Autodesk Inventor part; units mm, degrees
(part 2 of 2)
  spline S257 degree 2 poles (-118.3929, 389.4341) (-118.546, 389.3872) (-118.7461, 389.1921) (-118.7461, 389.0192) knots 0 0 0 1 2 2 2
  spline S258 degree 2 poles (-118.7461, 389.0192) (-118.7461, 388.8216) (-118.5238, 388.6215) (-118.3114, 388.6215) knots 0 0 0 1 2 2 2
  spline S259 degree 2 poles (-118.3114, 388.6215) (-118.1311, 388.6215) (-117.8347, 388.7771) (-117.7062, 388.8932) knots 0 0 0 1 2 2 2
  spline S260 degree 2 poles (-116.0884, 388.2856) (-116.402, 388.2856) (-116.7553, 388.6437) (-116.7553, 389.0315) knots 0 0 0 1 2 2 2
  line L211 (-116.7553, 389.0315) -> (-116.7553, 390.2986)
  line L212 (-116.7553, 390.2986) -> (-117.0146, 390.2986)
  line L213 (-117.0146, 390.2986) -> (-117.0146, 390.6173)
  line L214 (-117.0146, 390.6173) -> (-116.7553, 390.6173)
  line L215 (-116.7553, 390.6173) -> (-116.7553, 391.2743)
  line L216 (-116.7553, 391.2743) -> (-116.3699, 391.2743)
  line L217 (-116.3699, 391.2743) -> (-116.3699, 390.6173)
  line L218 (-116.3699, 390.6173) -> (-115.661, 390.6173)
  line L219 (-115.661, 390.6173) -> (-115.661, 390.2986)
  line L220 (-115.661, 390.2986) -> (-116.3699, 390.2986)
  line L221 (-116.3699, 390.2986) -> (-116.3699, 389.2094)
  spline S261 degree 2 poles (-116.3699, 389.2094) (-116.3699, 389.0365) (-116.3576, 388.8463) (-116.3156, 388.7648) knots 0 0 0 1 2 2 2
  spline S262 degree 2 poles (-116.3156, 388.7648) (-116.281, 388.6931) (-116.1254, 388.6215) (-115.992, 388.6215) knots 0 0 0 1 2 2 2
  spline S263 degree 2 poles (-115.992, 388.6215) (-115.8982, 388.6215) (-115.7228, 388.6783) (-115.6833, 388.6956) knots 0 0 0 1 2 2 2
  line L222 (-115.6833, 388.6956) -> (-115.661, 388.6956)
  line L223 (-115.661, 388.6956) -> (-115.661, 388.3498)
  spline S264 degree 2 poles (-115.661, 388.3498) (-115.7697, 388.3202) (-115.992, 388.2856) (-116.0884, 388.2856) knots 0 0 0 1 2 2 2
  spline S265 degree 2 poles (-114.384, 388.2782) (-114.9324, 388.2782) (-115.5351, 388.8932) (-115.5351, 389.4613) knots 0 0 0 1 2 2 2
  spline S266 degree 2 poles (-115.5351, 389.4613) (-115.5351, 390.0195) (-114.9497, 390.6815) (-114.4779, 390.6815) knots 0 0 0 1 2 2 2
  spline S267 degree 2 poles (-114.4779, 390.6815) (-114.2655, 390.6815) (-113.937, 390.558) (-113.8159, 390.4271) knots 0 0 0 1 2 2 2
  spline S268 degree 2 poles (-113.8159, 390.4271) (-113.6924, 390.2962) (-113.5615, 389.9183) (-113.5615, 389.6441) knots 0 0 0 1 2 2 2
  line L224 (-113.5615, 389.6441) -> (-113.5615, 389.4341)
  line L225 (-113.5615, 389.4341) -> (-115.1448, 389.4341)
  spline S269 degree 2 poles (-115.1448, 389.4341) (-115.1448, 389.0365) (-114.7447, 388.6141) (-114.389, 388.6141) knots 0 0 0 1 2 2 2
  spline S270 degree 2 poles (-114.389, 388.6141) (-114.263, 388.6141) (-114.0185, 388.6709) (-113.9197, 388.7154) knots 0 0 0 1 2 2 2
  spline S271 degree 2 poles (-113.9197, 388.7154) (-113.8159, 388.7648) (-113.6727, 388.8512) (-113.6257, 388.8907) knots 0 0 0 1 2 2 2
  line L226 (-113.6257, 388.8907) -> (-113.6035, 388.8907)
  line L227 (-113.6035, 388.8907) -> (-113.6035, 388.4708)
  spline S272 degree 2 poles (-113.6035, 388.4708) (-113.6702, 388.4437) (-113.8727, 388.3646) (-113.9518, 388.3424) knots 0 0 0 1 2 2 2
  spline S273 degree 2 poles (-113.9518, 388.3424) (-114.0629, 388.3103) (-114.2457, 388.2782) (-114.384, 388.2782) knots 0 0 0 1 2 2 2
  spline S274 degree 2 poles (-113.937, 389.7281) (-113.9419, 389.8837) (-114.0061, 390.1109) (-114.0679, 390.1875) knots 0 0 0 1 2 2 2
  spline S275 degree 2 poles (-114.0679, 390.1875) (-114.1346, 390.2739) (-114.3445, 390.3653) (-114.5001, 390.3653) knots 0 0 0 1 2 2 2
  spline S276 degree 2 poles (-114.5001, 390.3653) (-114.6533, 390.3653) (-114.8682, 390.2739) (-114.9571, 390.185) knots 0 0 0 1 2 2 2
  spline S277 degree 2 poles (-114.9571, 390.185) (-115.0435, 390.0936) (-115.1325, 389.8738) (-115.1448, 389.7281) knots 0 0 0 1 2 2 2
  line L228 (-115.1448, 389.7281) -> (-113.937, 389.7281)
  line L229 (-111.3756, 390.6173) -> (-112.2376, 388.33)
  line L230 (-112.2376, 388.33) -> (-112.5834, 388.33)
  line L231 (-112.5834, 388.33) -> (-113.438, 390.6173)
  line L232 (-113.438, 390.6173) -> (-113.0206, 390.6173)
  line L233 (-113.0206, 390.6173) -> (-112.3957, 388.8562)
  line L234 (-112.3957, 388.8562) -> (-111.7757, 390.6173)
  line L235 (-111.7757, 390.6173) -> (-111.3756, 390.6173)
  spline S278 degree 2 poles (-110.0912, 388.2782) (-110.6395, 388.2782) (-111.2422, 388.8932) (-111.2422, 389.4613) knots 0 0 0 1 2 2 2
  spline S279 degree 2 poles (-111.2422, 389.4613) (-111.2422, 390.0195) (-110.6568, 390.6815) (-110.185, 390.6815) knots 0 0 0 1 2 2 2
  spline S280 degree 2 poles (-110.185, 390.6815) (-109.9726, 390.6815) (-109.6441, 390.558) (-109.5231, 390.4271) knots 0 0 0 1 2 2 2
  spline S281 degree 2 poles (-109.5231, 390.4271) (-109.3995, 390.2962) (-109.2686, 389.9183) (-109.2686, 389.6441) knots 0 0 0 1 2 2 2
  line L236 (-109.2686, 389.6441) -> (-109.2686, 389.4341)
  line L237 (-109.2686, 389.4341) -> (-110.8519, 389.4341)
  spline S282 degree 2 poles (-110.8519, 389.4341) (-110.8519, 389.0365) (-110.4518, 388.6141) (-110.0961, 388.6141) knots 0 0 0 1 2 2 2
  spline S283 degree 2 poles (-110.0961, 388.6141) (-109.9701, 388.6141) (-109.7256, 388.6709) (-109.6268, 388.7154) knots 0 0 0 1 2 2 2
  spline S284 degree 2 poles (-109.6268, 388.7154) (-109.5231, 388.7648) (-109.3798, 388.8512) (-109.3329, 388.8907) knots 0 0 0 1 2 2 2
  line L238 (-109.3329, 388.8907) -> (-109.3106, 388.8907)
  line L239 (-109.3106, 388.8907) -> (-109.3106, 388.4708)
  spline S285 degree 2 poles (-109.3106, 388.4708) (-109.3773, 388.4437) (-109.5799, 388.3646) (-109.6589, 388.3424) knots 0 0 0 1 2 2 2
  spline S286 degree 2 poles (-109.6589, 388.3424) (-109.7701, 388.3103) (-109.9528, 388.2782) (-110.0912, 388.2782) knots 0 0 0 1 2 2 2
  spline S287 degree 2 poles (-109.6441, 389.7281) (-109.649, 389.8837) (-109.7132, 390.1109) (-109.775, 390.1875) knots 0 0 0 1 2 2 2
  spline S288 degree 2 poles (-109.775, 390.1875) (-109.8417, 390.2739) (-110.0516, 390.3653) (-110.2072, 390.3653) knots 0 0 0 1 2 2 2
  spline S289 degree 2 poles (-110.2072, 390.3653) (-110.3604, 390.3653) (-110.5753, 390.2739) (-110.6642, 390.185) knots 0 0 0 1 2 2 2
  spline S290 degree 2 poles (-110.6642, 390.185) (-110.7506, 390.0936) (-110.8396, 389.8738) (-110.8519, 389.7281) knots 0 0 0 1 2 2 2
  line L240 (-110.8519, 389.7281) -> (-109.6441, 389.7281)
  line L241 (-107.6656, 390.2048) -> (-107.6854, 390.2048)
  spline S291 degree 2 poles (-107.6854, 390.2048) (-107.7298, 390.2171) (-107.8261, 390.2221) (-107.8928, 390.2221) knots 0 0 0 1 2 2 2
  spline S292 degree 2 poles (-107.8928, 390.2221) (-108.0485, 390.2221) (-108.3547, 390.0862) (-108.4931, 389.9528) knots 0 0 0 1 2 2 2
  line L242 (-108.4931, 389.9528) -> (-108.4931, 388.33)
  line L243 (-108.4931, 388.33) -> (-108.8784, 388.33)
  line L244 (-108.8784, 388.33) -> (-108.8784, 390.6173)
  line L245 (-108.8784, 390.6173) -> (-108.4931, 390.6173)
  line L246 (-108.4931, 390.6173) -> (-108.4931, 390.2764)
  spline S293 degree 2 poles (-108.4931, 390.2764) (-108.2831, 390.4641) (-107.9694, 390.6173) (-107.8212, 390.6173) knots 0 0 0 1 2 2 2
  spline S294 degree 2 poles (-107.8212, 390.6173) (-107.7619, 390.6173) (-107.7026, 390.6123) (-107.6656, 390.6049) knots 0 0 0 1 2 2 2
  line L247 (-107.6656, 390.6049) -> (-107.6656, 390.2048)
  line L248 (-104.2619, 388.33) -> (-104.6472, 388.33)
  line L249 (-104.6472, 388.33) -> (-104.6472, 389.6342)
  spline S295 degree 2 poles (-104.6472, 389.6342) (-104.6472, 389.7923) (-104.6769, 390.064) (-104.7213, 390.1455) knots 0 0 0 1 2 2 2
  spline S296 degree 2 poles (-104.7213, 390.1455) (-104.7683, 390.232) (-104.9362, 390.3159) (-105.0795, 390.3159) knots 0 0 0 1 2 2 2
  spline S297 degree 2 poles (-105.0795, 390.3159) (-105.2228, 390.3159) (-105.5266, 390.1628) (-105.6723, 390.0393) knots 0 0 0 1 2 2 2
  line L250 (-105.6723, 390.0393) -> (-105.6723, 388.33)
  line L251 (-105.6723, 388.33) -> (-106.0576, 388.33)
  line L252 (-106.0576, 388.33) -> (-106.0576, 391.5139)
  line L253 (-106.0576, 391.5139) -> (-105.6723, 391.5139)
  line L254 (-105.6723, 391.5139) -> (-105.6723, 390.3629)
  spline S298 degree 2 poles (-105.6723, 390.3629) (-105.4994, 390.5185) (-105.1659, 390.6815) (-104.9782, 390.6815) knots 0 0 0 1 2 2 2
  spline S299 degree 2 poles (-104.9782, 390.6815) (-104.6423, 390.6815) (-104.2619, 390.2369) (-104.2619, 389.8145) knots 0 0 0 1 2 2 2
  line L255 (-104.2619, 389.8145) -> (-104.2619, 388.33)
  spline S300 degree 2 poles (-102.728, 388.2782) (-103.2764, 388.2782) (-103.8791, 388.8932) (-103.8791, 389.4613) knots 0 0 0 1 2 2 2
  spline S301 degree 2 poles (-103.8791, 389.4613) (-103.8791, 390.0195) (-103.2937, 390.6815) (-102.8219, 390.6815) knots 0 0 0 1 2 2 2
  spline S302 degree 2 poles (-102.8219, 390.6815) (-102.6095, 390.6815) (-102.281, 390.558) (-102.1599, 390.4271) knots 0 0 0 1 2 2 2
  spline S303 degree 2 poles (-102.1599, 390.4271) (-102.0364, 390.2962) (-101.9055, 389.9183) (-101.9055, 389.6441) knots 0 0 0 1 2 2 2
  line L256 (-101.9055, 389.6441) -> (-101.9055, 389.4341)
  line L257 (-101.9055, 389.4341) -> (-103.4888, 389.4341)
  spline S304 degree 2 poles (-103.4888, 389.4341) (-103.4888, 389.0365) (-103.0887, 388.6141) (-102.733, 388.6141) knots 0 0 0 1 2 2 2
  spline S305 degree 2 poles (-102.733, 388.6141) (-102.607, 388.6141) (-102.3625, 388.6709) (-102.2637, 388.7154) knots 0 0 0 1 2 2 2
  spline S306 degree 2 poles (-102.2637, 388.7154) (-102.1599, 388.7648) (-102.0167, 388.8512) (-101.9697, 388.8907) knots 0 0 0 1 2 2 2
  line L258 (-101.9697, 388.8907) -> (-101.9475, 388.8907)
  line L259 (-101.9475, 388.8907) -> (-101.9475, 388.4708)
  spline S307 degree 2 poles (-101.9475, 388.4708) (-102.0142, 388.4437) (-102.2167, 388.3646) (-102.2958, 388.3424) knots 0 0 0 1 2 2 2
  spline S308 degree 2 poles (-102.2958, 388.3424) (-102.4069, 388.3103) (-102.5897, 388.2782) (-102.728, 388.2782) knots 0 0 0 1 2 2 2
  spline S309 degree 2 poles (-102.281, 389.7281) (-102.2859, 389.8837) (-102.3501, 390.1109) (-102.4119, 390.1875) knots 0 0 0 1 2 2 2
  spline S310 degree 2 poles (-102.4119, 390.1875) (-102.4786, 390.2739) (-102.6885, 390.3653) (-102.8441, 390.3653) knots 0 0 0 1 2 2 2
  spline S311 degree 2 poles (-102.8441, 390.3653) (-102.9973, 390.3653) (-103.2122, 390.2739) (-103.3011, 390.185) knots 0 0 0 1 2 2 2
  spline S312 degree 2 poles (-103.3011, 390.185) (-103.3875, 390.0936) (-103.4765, 389.8738) (-103.4888, 389.7281) knots 0 0 0 1 2 2 2
  line L260 (-103.4888, 389.7281) -> (-102.281, 389.7281)
  line L261 (-100.3025, 390.2048) -> (-100.3222, 390.2048)
  spline S313 degree 2 poles (-100.3222, 390.2048) (-100.3667, 390.2171) (-100.463, 390.2221) (-100.5297, 390.2221) knots 0 0 0 1 2 2 2
  spline S314 degree 2 poles (-100.5297, 390.2221) (-100.6853, 390.2221) (-100.9916, 390.0862) (-101.1299, 389.9528) knots 0 0 0 1 2 2 2
  line L262 (-101.1299, 389.9528) -> (-101.1299, 388.33)
  line L263 (-101.1299, 388.33) -> (-101.5153, 388.33)
  line L264 (-101.5153, 388.33) -> (-101.5153, 390.6173)
  line L265 (-101.5153, 390.6173) -> (-101.1299, 390.6173)
  line L266 (-101.1299, 390.6173) -> (-101.1299, 390.2764)
  spline S315 degree 2 poles (-101.1299, 390.2764) (-100.92, 390.4641) (-100.6063, 390.6173) (-100.4581, 390.6173) knots 0 0 0 1 2 2 2
  spline S316 degree 2 poles (-100.4581, 390.6173) (-100.3988, 390.6173) (-100.3395, 390.6123) (-100.3025, 390.6049) knots 0 0 0 1 2 2 2
  line L267 (-100.3025, 390.6049) -> (-100.3025, 390.2048)
  spline S317 degree 2 poles (-99.0107, 388.2782) (-99.559, 388.2782) (-100.1617, 388.8932) (-100.1617, 389.4613) knots 0 0 0 1 2 2 2
  spline S318 degree 2 poles (-100.1617, 389.4613) (-100.1617, 390.0195) (-99.5763, 390.6815) (-99.1045, 390.6815) knots 0 0 0 1 2 2 2
  spline S319 degree 2 poles (-99.1045, 390.6815) (-98.8921, 390.6815) (-98.5636, 390.558) (-98.4426, 390.4271) knots 0 0 0 1 2 2 2
  spline S320 degree 2 poles (-98.4426, 390.4271) (-98.3191, 390.2962) (-98.1881, 389.9183) (-98.1881, 389.6441) knots 0 0 0 1 2 2 2
  line L268 (-98.1881, 389.6441) -> (-98.1881, 389.4341)
  line L269 (-98.1881, 389.4341) -> (-99.7714, 389.4341)
  spline S321 degree 2 poles (-99.7714, 389.4341) (-99.7714, 389.0365) (-99.3713, 388.6141) (-99.0156, 388.6141) knots 0 0 0 1 2 2 2
  spline S322 degree 2 poles (-99.0156, 388.6141) (-98.8896, 388.6141) (-98.6451, 388.6709) (-98.5463, 388.7154) knots 0 0 0 1 2 2 2
  spline S323 degree 2 poles (-98.5463, 388.7154) (-98.4426, 388.7648) (-98.2993, 388.8512) (-98.2524, 388.8907) knots 0 0 0 1 2 2 2
  line L270 (-98.2524, 388.8907) -> (-98.2301, 388.8907)
  line L271 (-98.2301, 388.8907) -> (-98.2301, 388.4708)
  spline S324 degree 2 poles (-98.2301, 388.4708) (-98.2968, 388.4437) (-98.4994, 388.3646) (-98.5784, 388.3424) knots 0 0 0 1 2 2 2
  spline S325 degree 2 poles (-98.5784, 388.3424) (-98.6896, 388.3103) (-98.8723, 388.2782) (-99.0107, 388.2782) knots 0 0 0 1 2 2 2
  spline S326 degree 2 poles (-98.5636, 389.7281) (-98.5685, 389.8837) (-98.6327, 390.1109) (-98.6945, 390.1875) knots 0 0 0 1 2 2 2
  spline S327 degree 2 poles (-98.6945, 390.1875) (-98.7612, 390.2739) (-98.9711, 390.3653) (-99.1268, 390.3653) knots 0 0 0 1 2 2 2
  spline S328 degree 2 poles (-99.1268, 390.3653) (-99.2799, 390.3653) (-99.4948, 390.2739) (-99.5837, 390.185) knots 0 0 0 1 2 2 2
  spline S329 degree 2 poles (-99.5837, 390.185) (-99.6702, 390.0936) (-99.7591, 389.8738) (-99.7714, 389.7281) knots 0 0 0 1 2 2 2
  line L272 (-99.7714, 389.7281) -> (-98.5636, 389.7281)
  point P0 (0, 0)
  constraints: 2 other
emboss "Emboss1" sketch "Sketch4" operation cut depth 50.8 direction (0, 0, 1)
body "Solid1"
